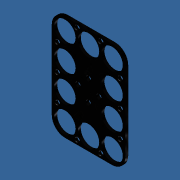
# Autodesk Inventor part: magnetic-mesh
Saved by Autodesk Inventor 2015 (Build 190159000, 159)
## iProperties
Created: 2019-02-02
Part Number: magnetic-mesh
Material: Generic
Document SubType Name: Modeling
Designer: gabriel
Density: 1 g/cm^3
Appearance: Default
Author: gabriel
Autodesk Inventor part; units mm, degrees
ref_plane "YZ Plane" through (0, 0, 0) normal (1, 0, 0) x (0, 1, 0)
ref_plane "XZ Plane" through (0, 0, 0) normal (0, 1, 0) x (-1, 0, 0)
ref_plane "XY Plane" through (0, 0, 0) normal (0, 0, 1) x (1, 0, 0)
sketch "Sketch27" plane through (0, 0, 0) normal (0, 0, 1) x (1, 0, 0)
  line L0 (0, -7.9375) -> (-28.575, -7.9375)
  line L1 (-36.5125, 0) -> (-36.5125, 47.625)
  line L2 (-28.575, 55.5625) -> (0, 55.5625)
  line L3 (7.9375, 47.625) -> (7.9375, 0)
  circle A0 centre (-28.575, 47.625) radius 6.4492
  circle A1 centre (-28.575, 31.75) radius 6.4492
  circle A2 centre (-28.575, 15.875) radius 6.4492
  circle A3 centre (-28.575, 0) radius 6.4492
  circle A4 centre (-14.2875, 0) radius 6.4492
  circle A5 centre (-14.2875, 47.625) radius 6.4492
  circle A6 centre (0, 47.625) radius 6.4492
  circle A7 centre (0, 31.75) radius 6.4492
  circle A8 centre (0, 15.875) radius 6.4492
  circle A9 centre (0, 0) radius 6.4492
  arc A10 (-28.575, 55.5625) -> (-36.5125, 47.625) centre (-28.575, 47.625) ccw
  arc A11 (7.9375, 47.625) -> (0, 55.5625) centre (0, 47.625) ccw
  arc A12 (-36.5125, 0) -> (-28.575, -7.9375) centre (-28.575, 0) ccw
  arc A13 (0, -7.9375) -> (7.9375, 0) centre (0, 0) ccw
  circle A14 centre (-33.3375, 39.6875) radius 1.3891
  circle A15 centre (-33.3375, 23.8125) radius 1.3891
  circle A16 centre (-33.3375, 7.9375) radius 1.3891
  circle A17 centre (4.7625, 39.6875) radius 1.3891
  circle A18 centre (4.7625, 23.8125) radius 1.3891
  circle A19 centre (4.7625, 7.9375) radius 1.3891
  circle A20 centre (-21.4312, 53.1812) radius 1.3891
  circle A21 centre (-7.1437, 53.1812) radius 1.3891
  circle A22 centre (-21.4312, -5.5562) radius 1.3891
  circle A23 centre (-7.1437, -5.5562) radius 1.3891
  dimension "d126" = 12.8984
  dimension "d127" = 12.8984
  dimension "d128" = 12.8984
  dimension "d129" = 12.8984
  dimension "d130" = 12.8984
  dimension "d131" = 12.8984
  dimension "d132" = 12.8984
  dimension "d133" = 12.8984
  dimension "d134" = 12.8984
  dimension "d135" = 12.8984
  dimension "d136" = 7.9375
  dimension "d137" = 14.2875
  dimension "d138" = 14.2875
  dimension "d139" = 7.9375
  dimension "d140" = 7.9375
  dimension "d141" = 15.875
  dimension "d142" = 15.875
  dimension "d145" = 44.45
  dimension "d146" = 63.5
  dimension "d149" = 2.7781
  dimension "d150" = 2.7781
  dimension "d151" = 2.7781
  dimension "d152" = 2.7781
  dimension "d153" = 2.7781
  dimension "d154" = 2.7781
  dimension "d155" = 3.175
  dimension "d156" = 3.175
  dimension "d157" = 15.875
  dimension "d158" = 15.875
  dimension "d159" = 15.875
  dimension "d162" = 2.7781
  dimension "d163" = 2.7781
  dimension "d164" = 2.7781
  dimension "d165" = 2.7781
  dimension "d166" = 2.3813
  dimension "d169" = 2.3813
  dimension "d170" = 7.1437
  dimension "d171" = 7.1437
  constraints: 24 centre point, 13 vertical alignment, 11 horizontal alignment, 8 end point, 8 point on circle, 5 coincident, 4 tangent, 2 parallel, 1 horizontal, 1 perpendicular
  measures "d126" diameter of A0
  measures "d127" diameter of A1
  measures "d128" diameter of A2
  measures "d129" diameter of A3
  measures "d130" diameter of A4
  measures "d131" diameter of A9
  measures "d132" diameter of A8
  measures "d133" diameter of A7
  measures "d134" diameter of A6
  measures "d135" diameter of A5
  measures "d136" distance from line of L1 A0.centre
  measures "d137" distance of A5.centre A0.centre
  measures "d138" distance of A5.centre A6.centre
  measures "d139" distance from line of L2 A0.centre
  measures "d140" distance from line of L0 A3.centre
  measures "d141" distance of A2.centre A3.centre
  measures "d142" distance of A0.centre A1.centre
  measures "d145" distance between parallel lines of L3 L1
  measures "d146" distance between parallel lines of L0 L2
  measures "d149" diameter of A14
  measures "d150" diameter of A15
  measures "d151" diameter of A16
  measures "d152" diameter of A17
  measures "d153" diameter of A18
  measures "d154" diameter of A19
  measures "d155" distance from line of L1 A14.centre
  measures "d156" distance from line of L3 A17.centre
  measures "d157" distance from line of L2 A14.centre
  measures "d158" distance of A15.centre A14.centre
  measures "d159" distance of A15.centre A16.centre
  measures "d162" diameter of A20
  measures "d163" diameter of A21
  measures "d164" diameter of A22
  measures "d165" diameter of A23
  measures "d166" distance from line of L2 A20.centre
  measures "d169" distance from line of L0 A22.centre
  measures "d170" horizontal distance of A10.centre A20.centre
  measures "d171" horizontal distance of A21.centre A5.centre
extrude "Extrusion26" add sketch "Sketch27" along normal blind 1.7859
fillet "Fillet1" radius 0.7937 10 edges at (-34.7266, 39.6875, 1.7859) (-34.7266, 23.8125, 1.7859) (-34.7266, 7.9375, 1.7859) (-22.8203, -5.5562, 1.7859) (-8.5328, -5.5562, 1.7859) (3.3734, 7.9375, 1.7859) (3.3734, 23.8125, 1.7859) (3.3734, 39.6875, 1.7859) (-8.5328, 53.1812, 1.7859) (-22.8203, 53.1812, 1.7859)
sketch "Sketch28" plane through (0, 0, 1.7859) normal (0, 0, 1) x (1, 0, 0)
  circle A0 centre (-14.2875, 30.1625) radius 1.5875
  circle A1 centre (-14.2875, 17.4625) radius 1.5875
  circle A2 centre (-7.9375, 23.8125) radius 1.5875
  circle A3 centre (-20.6375, 23.8125) radius 1.5875
  line L0 (7.9375, 0) -> (7.9375, 47.625) projected
  line L1 (-28.575, -7.9375) -> (0, -7.9375) projected
  point P0 (0, 0)
  dimension "d188" = 3.175
  dimension "d189" = 12.7
  dimension "d190" = 12.7
  dimension "d191" = 6.35
  dimension "d192" = 6.35
  dimension "d195" = 22.225
  dimension "d196" = 31.75
  constraints: 4 centre point, 3 equal radius, 1 horizontal alignment, 1 vertical alignment
  measures "d188" diameter of A0
  measures "d189" distance of A1.centre A0.centre
  measures "d190" distance of A2.centre A3.centre
  measures "d191" horizontal distance of A3.centre A0.centre
  measures "d192" horizontal distance of A3.centre A0.centre
  measures "d195" distance from line of L0 A1.centre
  measures "d196" distance from line of L1 A2.centre
extrude "Extrusion27" cut sketch "Sketch28" against normal through all
equation "\"d127\" = d126"
equation "\"d128\" = d126"
equation "\"d129\" = d126"
equation "\"d130\" = d126"
equation "\"d131\" = d126"
equation "\"d132\" = d126"
equation "\"d133\" = d126"
equation "\"d134\" = d126"
equation "\"d135\" = d126"
equation "\"d138\" = d137"
equation "\"d139\" = d136"
equation "\"d140\" = d136"
equation "\"d142\" = d141"
equation "\"d150\" = d149"
equation "\"d151\" = d149"
equation "\"d152\" = d149"
equation "\"d153\" = d149"
equation "\"d154\" = d149"
equation "\"d158\" = d157"
equation "\"d159\" = d157"
equation "\"d162\" = d149"
equation "\"d163\" = d149"
equation "\"d164\" = d149"
equation "\"d165\" = d149"
equation "\"d170\" = 0.5 * d137"
equation "\"d171\" = d170"
equation "\"d191\" = 0.5 * d190"
equation "\"d192\" = 0.5 * d189"
body "Solid10"
